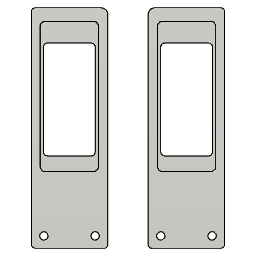
mriya-cnc-display-cover-v1.01 (Autodesk Fusion 360 design; units mm, degrees)
Autodesk Fusion 360 part; units mm, degrees
sketch "mriya-display-cover" plane through (0, 0, 0) normal (0, 0, 1) x (1, 0, 0)
  line L0 (-21.4, 23.7) -> (-21.4, 60.3)
  line L1 (-22.7, 5) -> (-5.8, 5) construction
  line L2 (-5, 5.8) -> (-5, 62) construction
  arc A0 (-5.8, 5) -> (-5, 5.8) centre (-5.8, 5.8) ccw construction
  arc A1 (-23.5, 5.8) -> (-22.7, 5) centre (-22.7, 5.8) ccw construction
  line L3 (-4.9, 5) -> (-4.9, 62)
  line L4 (-7.2, 60.3) -> (-7.2, 23.7)
  line L5 (-23.5, 5.8) -> (-23.5, 62.7) construction
  line L6 (-23.5, 63.6) -> (-6.5, 63.6)
  arc A2 (-10, 62.8) -> (-9.3, 63.5) centre (-10, 63.5) ccw construction
  line L7 (-20.6, 27.5) -> (-20.6, 55)
  line L8 (-8, 55) -> (-8, 27.5)
  arc A3 (-19.3, 63.5) -> (-18.6, 62.8) centre (-18.6, 63.5) ccw construction
  line L9 (-20.6, 55) -> (-8, 55)
  line L10 (-18.6, 62.8) -> (-10, 62.8) construction
  arc A4 (-22.7, 63.5) -> (-23.5, 62.7) centre (-22.7, 62.7) ccw construction
  line L11 (-22.7, 63.5) -> (-6.5, 63.5) construction
  line L12 (-21.4, 60.3) -> (-7.2, 60.3)
  line L13 (-20.6, 27.5) -> (-8, 27.5)
  line L14 (-23.5, 5) -> (-4.9, 5)
  circle A5 centre (-8, 8) radius 1.4
  circle A6 centre (-8, 20.7) radius 1 construction
  circle A7 centre (-20.5, 8) radius 1.4
  line L15 (-23.5, 5) -> (-23.5, 63.6)
  arc A8 (-5, 62) -> (-6.5, 63.5) centre (-6.5, 62) ccw construction
  arc A9 (-4.9, 62) -> (-6.5, 63.6) centre (-6.5, 62) ccw
  circle A10 centre (-20.5, 8) radius 1
  circle A11 centre (-8, 8) radius 1
  line L16 (-21.4, 23.7) -> (-7.2, 23.7)
  line L17 (-5, 23.7) -> (-4.9, 23.7)
  dimension "d601" = 2.8
  dimension "d602" = 2.8
  dimension "d606" = 2
  dimension "d609" = 2
  dimension "d610" = 2
  constraint perpendicular L2 L11
  constraint perpendicular L1 L5
  constraint tangent A1 L5
  constraint tangent L1 A1
  constraint tangent L2 A0
  constraint tangent L1 A0
  constraint tangent L5 A4
  constraint tangent A4 L11
  constraint tangent L2 A8
  constraint tangent L11 A8
  constraint perpendicular L7 L13
  constraint perpendicular L7 L9
  constraint perpendicular L8 L13
  constraint coincident L17.end L3
  constraint perpendicular L3 L14
  constraint perpendicular L6 L15
  constraint tangent A3 L10
  constraint tangent A2 L10
  constraint tangent L6 A9
  constraint tangent L3 A9
  constraint concentric A7 A10
  constraint concentric A5 A11
  constraint coincident L2 L17.start
  constraint collinear L16 L17
  measures "d601" diameter of A7
  measures "d602" diameter of A5
  measures "d606" diameter of A6
  measures "d609" diameter of A10
  measures "d610" diameter of A11
extrude "Extrude78" add sketch "mriya-display-cover" along normal blind 1.5 contours L3 L6 L14 L15 A9 makes body 1
extrude "Extrude79" add sketch "mriya-display-cover" along normal blind 0.7 contours L0 L4 L12 L16 bodies 1
extrude "Extrude80" add sketch "mriya-display-cover" along normal blind 0.7 from surface at 0.8 contours A5 | A7 bodies 1
fillet "Fillet57" radius 0.8 3 edges at (-4.9, 5, 0.75) (-23.5, 5, 0.75) (-23.5, 63.6, 0.75) on bodies 1
fillet "Fillet58" radius 1 4 edges at (-20.6, 27.5, 0.35) (-8, 27.5, 0.35) (-20.6, 55, 0.35) (-8, 55, 0.35) on bodies 1
fillet "Fillet59" radius 1.2 4 edges at (-7.2, 23.7, 1.1) (-21.4, 23.7, 1.1) (-21.4, 60.3, 1.1) (-7.2, 60.3, 1.1) on bodies 1
mirror "Mirror10" about plane through (0, 0, 0) normal (1, 0, 0) of bodies 1 makes body 2
named bodies: "Right", "Left"
